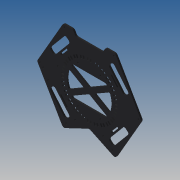
# Autodesk Inventor part: Bottom Plate
Saved by Autodesk Inventor 2017 (Build 210142000, 142)
## iProperties
Created: 2016-10-01
Part Number: Bottom Plate
Material: PVC, Unplasticized
Document SubType Name: Modeling
Designer: James Yelland
Density: 1.29 g/cm^3
Appearance: Smooth - White
Mass: 43.6601 g
Surface Area: 401.333 cm^2
Volume: 33.8451 cm^3
Author: James Yelland
Autodesk Inventor part; units mm, degrees
ref_plane "YZ Plane" through (0, 0, 0) normal (1, 0, 0) x (0, 1, 0)
ref_plane "XZ Plane" through (0, 0, 0) normal (0, 1, 0) x (-1, 0, 0)
ref_plane "XY Plane" through (0, 0, 0) normal (0, 0, 1) x (1, 0, 0)
sketch "Sketch1" plane through (0, 0, 0) normal (0, 1, 0) x (-1, 0, 0)
  line L0 (103.5566, -2.5) -> (54.7862, -86.9325)
  line L1 (-54.8095, -86.9325) -> (-103.5566, -2.5)
  line L2 (-103.5566, 2.5) -> (-53.9434, 88.4327)
  line L3 (53.9434, 88.4327) -> (103.5566, 2.5)
  line L4 (2.1497, -66.9563) -> (48.3064, -88.9468)
  line L5 (-2.1497, -66.9563) -> (-48.3297, -88.9468)
  arc A0 (48.3064, -88.9468) -> (54.7862, -86.9325) centre (50.456, -84.4325) ccw
  arc A1 (2.1497, -66.9563) -> (-2.1497, -66.9563) centre (0, -71.4706) ccw
  arc A2 (-54.8095, -86.9325) -> (-48.3297, -88.9468) centre (-50.4794, -84.4325) ccw
  arc A3 (-103.5566, 2.5) -> (-103.5566, -2.5) centre (-99.2265, 0) ccw
  arc A4 (-49.6132, 90.9327) -> (-53.9434, 88.4327) centre (-49.6132, 85.9327) ccw
  arc A5 (53.9434, 88.4327) -> (49.6132, 90.9327) centre (49.6132, 85.9327) ccw
  arc A6 (103.5566, -2.5) -> (103.5566, 2.5) centre (99.2265, 0) ccw
  circle A7 centre (49.6132, 85.9327) radius 1.6
  circle A8 centre (-49.6132, 85.9327) radius 1.6
  circle A9 centre (-99.2265, 0) radius 1.6
  circle A10 centre (99.2265, 0) radius 1.6
  line L6 (1.5, -53.75) -> (1.5, -56.75)
  line L7 (1.5, -56.75) -> (4.5, -56.75)
  line L8 (4.5, -56.75) -> (4.5, -50.75)
  line L9 (4.5, -50.75) -> (1.5, -50.75)
  line L10 (1.5, -50.75) -> (1.5, -53.75)
  line L11 (-1.5, -53.75) -> (-1.5, -56.75)
  line L12 (-1.5, -56.75) -> (-4.5, -56.75)
  line L13 (-1.5, -53.75) -> (-1.5, -53.75)
  line L14 (-1.5, -53.75) -> (-1.5, -50.75)
  line L15 (-1.5, -50.75) -> (-4.5, -50.75)
  line L16 (-4.5, -56.75) -> (-4.5, -50.75)
  line L17 (15.3604, -51.5303) -> (16.1369, -54.4281)
  line L18 (16.1369, -54.4281) -> (19.0346, -53.6516)
  line L19 (19.0346, -53.6516) -> (17.4817, -47.856)
  line L20 (17.4817, -47.856) -> (14.584, -48.6325)
  line L21 (14.584, -48.6325) -> (15.3604, -51.5303)
  line L22 (12.4626, -52.3067) -> (13.2391, -55.2045)
  line L23 (13.2391, -55.2045) -> (10.3413, -55.981)
  line L24 (12.4626, -52.3067) -> (11.6862, -49.409)
  line L25 (11.6862, -49.409) -> (8.7884, -50.1854)
  line L26 (10.3413, -55.981) -> (8.7884, -50.1854)
  line L27 (28.174, -45.7989) -> (29.674, -48.3969)
  line L28 (29.674, -48.3969) -> (32.2721, -46.8969)
  line L29 (32.2721, -46.8969) -> (29.2721, -41.7008)
  line L30 (29.2721, -41.7008) -> (26.674, -43.2008)
  line L31 (26.674, -43.2008) -> (28.174, -45.7989)
  line L32 (25.576, -47.2989) -> (27.076, -49.8969)
  line L33 (27.076, -49.8969) -> (24.4779, -51.3969)
  line L34 (25.576, -47.2989) -> (24.076, -44.7008)
  line L35 (24.076, -44.7008) -> (21.4779, -46.2008)
  line L36 (24.4779, -51.3969) -> (21.4779, -46.2008)
  line L37 (39.0676, -36.9463) -> (41.189, -39.0676)
  line L38 (41.189, -39.0676) -> (43.3103, -36.9463)
  line L39 (43.3103, -36.9463) -> (39.0676, -32.7037)
  line L40 (39.0676, -32.7037) -> (36.9463, -34.825)
  line L41 (36.9463, -34.825) -> (39.0676, -36.9463)
  line L42 (36.9463, -39.0676) -> (39.0676, -41.189)
  line L43 (39.0676, -41.189) -> (36.9463, -43.3103)
  line L44 (36.9463, -39.0676) -> (34.825, -36.9463)
  line L45 (34.825, -36.9463) -> (32.7037, -39.0676)
  line L46 (36.9463, -43.3103) -> (32.7037, -39.0676)
  line L47 (47.2989, -25.576) -> (49.8969, -27.076)
  line L48 (49.8969, -27.076) -> (51.3969, -24.4779)
  line L49 (51.3969, -24.4779) -> (46.2008, -21.4779)
  line L50 (46.2008, -21.4779) -> (44.7008, -24.076)
  line L51 (44.7008, -24.076) -> (47.2989, -25.576)
  line L52 (45.7989, -28.174) -> (48.3969, -29.674)
  line L53 (48.3969, -29.674) -> (46.8969, -32.2721)
  line L54 (45.7989, -28.174) -> (43.2008, -26.674)
  line L55 (43.2008, -26.674) -> (41.7008, -29.2721)
  line L56 (46.8969, -32.2721) -> (41.7008, -29.2721)
  line L57 (52.3067, -12.4626) -> (55.2045, -13.2391)
  line L58 (55.2045, -13.2391) -> (55.981, -10.3413)
  line L59 (55.981, -10.3413) -> (50.1854, -8.7884)
  line L60 (50.1854, -8.7884) -> (49.409, -11.6862)
  line L61 (49.409, -11.6862) -> (52.3067, -12.4626)
  line L62 (51.5303, -15.3604) -> (54.4281, -16.1369)
  line L63 (54.4281, -16.1369) -> (53.6516, -19.0346)
  line L64 (51.5303, -15.3604) -> (48.6325, -14.584)
  line L65 (48.6325, -14.584) -> (47.856, -17.4817)
  line L66 (53.6516, -19.0346) -> (47.856, -17.4817)
  line L67 (53.75, 1.5) -> (56.75, 1.5)
  line L68 (56.75, 1.5) -> (56.75, 4.5)
  line L69 (56.75, 4.5) -> (50.75, 4.5)
  line L70 (50.75, 4.5) -> (50.75, 1.5)
  line L71 (50.75, 1.5) -> (53.75, 1.5)
  line L72 (53.75, -1.5) -> (56.75, -1.5)
  line L73 (56.75, -1.5) -> (56.75, -4.5)
  line L74 (53.75, -1.5) -> (50.75, -1.5)
  line L75 (50.75, -1.5) -> (50.75, -4.5)
  line L76 (56.75, -4.5) -> (50.75, -4.5)
  line L77 (51.5303, 15.3604) -> (54.4281, 16.1369)
  line L78 (54.4281, 16.1369) -> (53.6516, 19.0346)
  line L79 (53.6516, 19.0346) -> (47.856, 17.4817)
  line L80 (47.856, 17.4817) -> (48.6325, 14.584)
  line L81 (48.6325, 14.584) -> (51.5303, 15.3604)
  line L82 (52.3067, 12.4626) -> (55.2045, 13.2391)
  line L83 (55.2045, 13.2391) -> (55.981, 10.3413)
  line L84 (52.3067, 12.4626) -> (49.409, 11.6862)
  line L85 (49.409, 11.6862) -> (50.1854, 8.7884)
  line L86 (55.981, 10.3413) -> (50.1854, 8.7884)
  line L87 (45.7989, 28.174) -> (48.3969, 29.674)
  line L88 (48.3969, 29.674) -> (46.8969, 32.2721)
  line L89 (46.8969, 32.2721) -> (41.7008, 29.2721)
  line L90 (41.7008, 29.2721) -> (43.2008, 26.674)
  line L91 (43.2008, 26.674) -> (45.7989, 28.174)
  line L92 (47.2989, 25.576) -> (49.8969, 27.076)
  line L93 (49.8969, 27.076) -> (51.3969, 24.4779)
  line L94 (47.2989, 25.576) -> (44.7008, 24.076)
  line L95 (44.7008, 24.076) -> (46.2008, 21.4779)
  line L96 (51.3969, 24.4779) -> (46.2008, 21.4779)
  line L97 (36.9463, 39.0676) -> (39.0676, 41.189)
  line L98 (39.0676, 41.189) -> (36.9463, 43.3103)
  line L99 (36.9463, 43.3103) -> (32.7037, 39.0676)
  line L100 (32.7037, 39.0676) -> (34.825, 36.9463)
  line L101 (34.825, 36.9463) -> (36.9463, 39.0676)
  line L102 (39.0676, 36.9463) -> (41.189, 39.0676)
  line L103 (41.189, 39.0676) -> (43.3103, 36.9463)
  line L104 (39.0676, 36.9463) -> (36.9463, 34.825)
  line L105 (36.9463, 34.825) -> (39.0676, 32.7037)
  line L106 (43.3103, 36.9463) -> (39.0676, 32.7037)
  line L107 (25.576, 47.2989) -> (27.076, 49.8969)
  line L108 (27.076, 49.8969) -> (24.4779, 51.3969)
  line L109 (24.4779, 51.3969) -> (21.4779, 46.2008)
  line L110 (21.4779, 46.2008) -> (24.076, 44.7008)
  line L111 (24.076, 44.7008) -> (25.576, 47.2989)
  line L112 (28.174, 45.7989) -> (29.674, 48.3969)
  line L113 (29.674, 48.3969) -> (32.2721, 46.8969)
  line L114 (28.174, 45.7989) -> (26.674, 43.2008)
  line L115 (26.674, 43.2008) -> (29.2721, 41.7008)
  line L116 (32.2721, 46.8969) -> (29.2721, 41.7008)
  line L117 (12.4626, 52.3067) -> (13.2391, 55.2045)
  line L118 (13.2391, 55.2045) -> (10.3413, 55.981)
  line L119 (10.3413, 55.981) -> (8.7884, 50.1854)
  line L120 (8.7884, 50.1854) -> (11.6862, 49.409)
  line L121 (11.6862, 49.409) -> (12.4626, 52.3067)
  line L122 (15.3604, 51.5303) -> (16.1369, 54.4281)
  line L123 (16.1369, 54.4281) -> (19.0346, 53.6516)
  line L124 (15.3604, 51.5303) -> (14.584, 48.6325)
  line L125 (14.584, 48.6325) -> (17.4817, 47.856)
  line L126 (19.0346, 53.6516) -> (17.4817, 47.856)
  line L127 (-1.5, 53.75) -> (-1.5, 56.75)
  line L128 (-1.5, 56.75) -> (-4.5, 56.75)
  line L129 (-4.5, 56.75) -> (-4.5, 50.75)
  line L130 (-4.5, 50.75) -> (-1.5, 50.75)
  line L131 (-1.5, 50.75) -> (-1.5, 53.75)
  line L132 (1.5, 53.75) -> (1.5, 56.75)
  line L133 (1.5, 56.75) -> (4.5, 56.75)
  line L134 (1.5, 53.75) -> (1.5, 50.75)
  line L135 (1.5, 50.75) -> (4.5, 50.75)
  line L136 (4.5, 56.75) -> (4.5, 50.75)
  line L137 (-15.3604, 51.5303) -> (-16.1369, 54.4281)
  line L138 (-16.1369, 54.4281) -> (-19.0346, 53.6516)
  line L139 (-19.0346, 53.6516) -> (-17.4817, 47.856)
  line L140 (-17.4817, 47.856) -> (-14.584, 48.6325)
  line L141 (-14.584, 48.6325) -> (-15.3604, 51.5303)
  line L142 (-12.4626, 52.3067) -> (-13.2391, 55.2045)
  line L143 (-13.2391, 55.2045) -> (-10.3413, 55.981)
  line L144 (-12.4626, 52.3067) -> (-11.6862, 49.409)
  line L145 (-11.6862, 49.409) -> (-8.7884, 50.1854)
  line L146 (-10.3413, 55.981) -> (-8.7884, 50.1854)
  line L147 (-28.174, 45.7989) -> (-29.674, 48.3969)
  line L148 (-29.674, 48.3969) -> (-32.2721, 46.8969)
  line L149 (-32.2721, 46.8969) -> (-29.2721, 41.7008)
  line L150 (-29.2721, 41.7008) -> (-26.674, 43.2008)
  line L151 (-26.674, 43.2008) -> (-28.174, 45.7989)
  line L152 (-25.576, 47.2989) -> (-27.076, 49.8969)
  line L153 (-27.076, 49.8969) -> (-24.4779, 51.3969)
  line L154 (-25.576, 47.2989) -> (-24.076, 44.7008)
  line L155 (-24.076, 44.7008) -> (-21.4779, 46.2008)
  line L156 (-24.4779, 51.3969) -> (-21.4779, 46.2008)
  line L157 (-39.0676, 36.9463) -> (-41.189, 39.0676)
  line L158 (-41.189, 39.0676) -> (-43.3103, 36.9463)
  line L159 (-43.3103, 36.9463) -> (-39.0676, 32.7037)
  line L160 (-39.0676, 32.7037) -> (-36.9463, 34.825)
  line L161 (-36.9463, 34.825) -> (-39.0676, 36.9463)
  line L162 (-36.9463, 39.0676) -> (-39.0676, 41.189)
  line L163 (-39.0676, 41.189) -> (-36.9463, 43.3103)
  line L164 (-36.9463, 39.0676) -> (-34.825, 36.9463)
  line L165 (-34.825, 36.9463) -> (-32.7037, 39.0676)
  line L166 (-36.9463, 43.3103) -> (-32.7037, 39.0676)
  line L167 (-47.2989, 25.576) -> (-49.8969, 27.076)
  line L168 (-49.8969, 27.076) -> (-51.3969, 24.4779)
  line L169 (-51.3969, 24.4779) -> (-46.2008, 21.4779)
  line L170 (-46.2008, 21.4779) -> (-44.7008, 24.076)
  line L171 (-44.7008, 24.076) -> (-47.2989, 25.576)
  line L172 (-45.7989, 28.174) -> (-48.3969, 29.674)
  line L173 (-48.3969, 29.674) -> (-46.8969, 32.2721)
  line L174 (-45.7989, 28.174) -> (-43.2008, 26.674)
  line L175 (-43.2008, 26.674) -> (-41.7008, 29.2721)
  line L176 (-46.8969, 32.2721) -> (-41.7008, 29.2721)
  line L177 (-52.3067, 12.4626) -> (-55.2045, 13.2391)
  line L178 (-55.2045, 13.2391) -> (-55.981, 10.3413)
  line L179 (-55.981, 10.3413) -> (-50.1854, 8.7884)
  line L180 (-50.1854, 8.7884) -> (-49.409, 11.6862)
  line L181 (-49.409, 11.6862) -> (-52.3067, 12.4626)
  line L182 (-51.5303, 15.3604) -> (-54.4281, 16.1369)
  line L183 (-54.4281, 16.1369) -> (-53.6516, 19.0346)
  line L184 (-51.5303, 15.3604) -> (-48.6325, 14.584)
  line L185 (-48.6325, 14.584) -> (-47.856, 17.4817)
  line L186 (-53.6516, 19.0346) -> (-47.856, 17.4817)
  line L187 (-53.75, -1.5) -> (-56.75, -1.5)
  line L188 (-56.75, -1.5) -> (-56.75, -4.5)
  line L189 (-56.75, -4.5) -> (-50.75, -4.5)
  line L190 (-50.75, -4.5) -> (-50.75, -1.5)
  line L191 (-50.75, -1.5) -> (-53.75, -1.5)
  line L192 (-53.75, 1.5) -> (-56.75, 1.5)
  line L193 (-56.75, 1.5) -> (-56.75, 4.5)
  line L194 (-53.75, 1.5) -> (-50.75, 1.5)
  line L195 (-50.75, 1.5) -> (-50.75, 4.5)
  line L196 (-56.75, 4.5) -> (-50.75, 4.5)
  line L197 (-51.5303, -15.3604) -> (-54.4281, -16.1369)
  line L198 (-54.4281, -16.1369) -> (-53.6516, -19.0346)
  line L199 (-53.6516, -19.0346) -> (-47.856, -17.4817)
  line L200 (-47.856, -17.4817) -> (-48.6325, -14.584)
  line L201 (-48.6325, -14.584) -> (-51.5303, -15.3604)
  line L202 (-52.3067, -12.4626) -> (-55.2045, -13.2391)
  line L203 (-55.2045, -13.2391) -> (-55.981, -10.3413)
  line L204 (-52.3067, -12.4626) -> (-49.409, -11.6862)
  line L205 (-49.409, -11.6862) -> (-50.1854, -8.7884)
  line L206 (-55.981, -10.3413) -> (-50.1854, -8.7884)
  line L207 (-45.7989, -28.174) -> (-48.3969, -29.674)
  line L208 (-48.3969, -29.674) -> (-46.8969, -32.2721)
  line L209 (-46.8969, -32.2721) -> (-41.7008, -29.2721)
  line L210 (-41.7008, -29.2721) -> (-43.2008, -26.674)
  line L211 (-43.2008, -26.674) -> (-45.7989, -28.174)
  line L212 (-47.2989, -25.576) -> (-49.8969, -27.076)
  line L213 (-49.8969, -27.076) -> (-51.3969, -24.4779)
  line L214 (-47.2989, -25.576) -> (-44.7008, -24.076)
  line L215 (-44.7008, -24.076) -> (-46.2008, -21.4779)
  line L216 (-51.3969, -24.4779) -> (-46.2008, -21.4779)
  line L217 (-36.9463, -39.0676) -> (-39.0676, -41.189)
  line L218 (-39.0676, -41.189) -> (-36.9463, -43.3103)
  line L219 (-36.9463, -43.3103) -> (-32.7037, -39.0676)
  line L220 (-32.7037, -39.0676) -> (-34.825, -36.9463)
  line L221 (-34.825, -36.9463) -> (-36.9463, -39.0676)
  line L222 (-39.0676, -36.9463) -> (-41.189, -39.0676)
  line L223 (-41.189, -39.0676) -> (-43.3103, -36.9463)
  line L224 (-39.0676, -36.9463) -> (-36.9463, -34.825)
  line L225 (-36.9463, -34.825) -> (-39.0676, -32.7037)
  line L226 (-43.3103, -36.9463) -> (-39.0676, -32.7037)
  line L227 (-25.576, -47.2989) -> (-27.076, -49.8969)
  line L228 (-27.076, -49.8969) -> (-24.4779, -51.3969)
  line L229 (-24.4779, -51.3969) -> (-21.4779, -46.2008)
  line L230 (-21.4779, -46.2008) -> (-24.076, -44.7008)
  line L231 (-24.076, -44.7008) -> (-25.576, -47.2989)
  line L232 (-28.174, -45.7989) -> (-29.674, -48.3969)
  line L233 (-29.674, -48.3969) -> (-32.2721, -46.8969)
  line L234 (-28.174, -45.7989) -> (-26.674, -43.2008)
  line L235 (-26.674, -43.2008) -> (-29.2721, -41.7008)
  line L236 (-32.2721, -46.8969) -> (-29.2721, -41.7008)
  line L237 (-12.4626, -52.3067) -> (-13.2391, -55.2045)
  line L238 (-13.2391, -55.2045) -> (-10.3413, -55.981)
  line L239 (-10.3413, -55.981) -> (-8.7884, -50.1854)
  line L240 (-8.7884, -50.1854) -> (-11.6862, -49.409)
  line L241 (-11.6862, -49.409) -> (-12.4626, -52.3067)
  line L242 (-15.3604, -51.5303) -> (-16.1369, -54.4281)
  line L243 (-16.1369, -54.4281) -> (-19.0346, -53.6516)
  line L244 (-15.3604, -51.5303) -> (-14.584, -48.6325)
  line L245 (-14.584, -48.6325) -> (-17.4817, -47.856)
  line L246 (-19.0346, -53.6516) -> (-17.4817, -47.856)
  arc A11 (50.7976, 70.0378) -> (45.1623, 70.5308) centre (47.7335, 67.4666) ccw
  line L247 (45.1623, 70.5308) -> (41.3321, 67.3169)
  arc A12 (41.3321, 67.3169) -> (40.8391, 61.6815) centre (43.9032, 64.2527) ccw
  line L248 (64.2962, 53.9509) -> (50.7976, 70.0378)
  line L249 (40.8391, 61.6815) -> (67.8361, 29.5077)
  line L250 (64.2962, 53.9509) -> (77.7947, 37.8639)
  arc A13 (77.3017, 32.2286) -> (77.7947, 37.8639) centre (74.7305, 35.2928) ccw
  line L251 (73.4714, 29.0147) -> (77.3017, 32.2286)
  arc A14 (67.8361, 29.5077) -> (73.4714, 29.0147) centre (70.9003, 32.0789) ccw
  line L252 (0, 30) -> (-31.225, 30)
  line L253 (0, 30) -> (31.225, 30)
  line L254 (0, -30) -> (-31.225, -30)
  line L255 (0, -30) -> (31.225, -30)
  arc A15 (42.1141, -15.8557) -> (42.1141, 15.8557) centre (0, 0) ccw
  arc A16 (-42.1141, 15.8558) -> (-42.1141, -15.8558) centre (0, 0) ccw
  arc A17 (34.525, 28.7563) -> (31.225, 30) centre (31.225, 25) ccw
  arc A18 (-31.225, 30) -> (-34.525, 28.7563) centre (-31.225, 25) ccw
  arc A19 (-34.525, -28.7563) -> (-31.225, -30) centre (-31.225, -25) ccw
  arc A20 (31.225, -30) -> (34.525, -28.7563) centre (31.225, -25) ccw
  circle A21 centre (22.6343, 38) radius 1.6
  circle A22 centre (-22.6343, 38) radius 1.6
  circle A23 centre (-22.6343, -38) radius 1.6
  circle A24 centre (22.6343, -38) radius 1.6
  line L256 (54.3376, 45.5946) -> (57.5515, 41.7644)
  line L257 (39.2424, -16.8831) -> (13, -1.7321)
  line L258 (39.2424, 16.8831) -> (13, 1.7321)
  line L259 (34.205, 25.5218) -> (1, 6.3509)
  line L260 (-1, 6.3509) -> (-34.205, 25.5218)
  line L261 (-39.2423, 16.8832) -> (-12.9998, 1.7321)
  line L262 (-12.9998, -1.7321) -> (-39.2423, -16.8832)
  line L263 (-34.205, -25.5218) -> (-1, -6.3509)
  line L264 (1, -6.3509) -> (34.205, -25.5218)
  arc A25 (-1, 6.3509) -> (1, 6.3509) centre (0, 8.0829) ccw
  arc A26 (-12.9998, -1.7321) -> (-12.9998, 1.7321) centre (-13.9998, 0) ccw
  arc A27 (1, -6.3509) -> (-1, -6.3509) centre (0, -8.0829) ccw
  arc A28 (13, 1.7321) -> (13, -1.7321) centre (14, 0) ccw
  arc A29 (39.2424, -16.8831) -> (42.1141, -15.8557) centre (40.2424, -15.151) ccw
  arc A30 (34.525, -28.7563) -> (34.205, -25.5218) centre (33.205, -27.2538) ccw
  arc A31 (-42.1141, -15.8558) -> (-39.2423, -16.8832) centre (-40.2423, -15.1511) ccw
  arc A32 (-34.205, -25.5218) -> (-34.525, -28.7563) centre (-33.205, -27.2538) ccw
  arc A33 (-39.2423, 16.8832) -> (-42.1141, 15.8558) centre (-40.2423, 15.1511) ccw
  arc A34 (-34.525, 28.7563) -> (-34.205, 25.5218) centre (-33.205, 27.2538) ccw
  arc A35 (42.1141, 15.8557) -> (39.2424, 16.8831) centre (40.2424, 15.151) ccw
  arc A36 (34.205, 25.5218) -> (34.525, 28.7563) centre (33.205, 27.2538) ccw
  line L265 (49.7796, 41.77) -> (43.3517, 49.4305)
  line L266 (43.3517, 49.4305) -> (45.6499, 51.3589)
  line L267 (45.6499, 51.3589) -> (58.5056, 36.038)
  line L268 (58.5056, 36.038) -> (56.2075, 34.1096)
  line L269 (56.2075, 34.1096) -> (49.7796, 41.77)
  arc A37 (73.4714, -29.0147) -> (67.8361, -29.5077) centre (70.9003, -32.0789) ccw
  arc A38 (77.7947, -37.8639) -> (77.3017, -32.2286) centre (74.7305, -35.2928) ccw
  line L270 (73.4714, -29.0147) -> (77.3017, -32.2286)
  arc A39 (45.1623, -70.5308) -> (50.7976, -70.0378) centre (47.7335, -67.4666) ccw
  line L271 (45.1623, -70.5308) -> (41.3321, -67.3169)
  arc A40 (40.8391, -61.6815) -> (41.3321, -67.3169) centre (43.9032, -64.2527) ccw
  line L272 (64.2962, -53.9509) -> (50.7976, -70.0378)
  line L273 (64.2962, -53.9509) -> (77.7947, -37.8639)
  line L274 (40.8391, -61.6815) -> (67.8361, -29.5077)
  line L275 (49.7796, -41.77) -> (43.3517, -49.4305)
  line L276 (43.3517, -49.4305) -> (45.6499, -51.3589)
  line L277 (45.6499, -51.3589) -> (58.5056, -36.038)
  line L278 (58.5056, -36.038) -> (56.2075, -34.1096)
  line L279 (56.2075, -34.1096) -> (49.7796, -41.77)
  arc A41 (-73.4714, 29.0147) -> (-67.8361, 29.5077) centre (-70.9003, 32.0789) ccw
  arc A42 (-77.7947, 37.8639) -> (-77.3017, 32.2286) centre (-74.7305, 35.2928) ccw
  line L280 (-73.4714, 29.0147) -> (-77.3017, 32.2286)
  arc A43 (-45.1623, 70.5308) -> (-50.7976, 70.0378) centre (-47.7335, 67.4666) ccw
  line L281 (-45.1623, 70.5308) -> (-41.3321, 67.3169)
  arc A44 (-40.8391, 61.6815) -> (-41.3321, 67.3169) centre (-43.9032, 64.2527) ccw
  line L282 (-64.2962, 53.9509) -> (-50.7976, 70.0378)
  line L283 (-64.2962, 53.9509) -> (-77.7947, 37.8639)
  line L284 (-40.8391, 61.6815) -> (-67.8361, 29.5077)
  line L285 (-49.7796, 41.77) -> (-43.3517, 49.4305)
  line L286 (-43.3517, 49.4305) -> (-45.6499, 51.3589)
  line L287 (-45.6499, 51.3589) -> (-58.5056, 36.038)
  line L288 (-58.5056, 36.038) -> (-56.2075, 34.1096)
  line L289 (-56.2075, 34.1096) -> (-49.7796, 41.77)
  arc A45 (-67.8361, -29.5077) -> (-73.4714, -29.0147) centre (-70.9003, -32.0789) ccw
  line L290 (-45.6499, -51.3589) -> (-58.5056, -36.038)
  line L291 (-58.5056, -36.038) -> (-56.2075, -34.1096)
  line L292 (-40.8391, -61.6815) -> (-67.8361, -29.5077)
  line L293 (-64.2962, -53.9509) -> (-77.7947, -37.8639)
  line L294 (-73.4714, -29.0147) -> (-77.3017, -32.2286)
  arc A46 (-77.3017, -32.2286) -> (-77.7947, -37.8639) centre (-74.7305, -35.2928) ccw
  line L295 (-43.3517, -49.4305) -> (-45.6499, -51.3589)
  line L296 (-49.7796, -41.77) -> (-43.3517, -49.4305)
  arc A47 (-50.7976, -70.0378) -> (-45.1623, -70.5308) centre (-47.7335, -67.4666) ccw
  line L297 (-64.2962, -53.9509) -> (-50.7976, -70.0378)
  line L298 (-45.1623, -70.5308) -> (-41.3321, -67.3169)
  arc A48 (-41.3321, -67.3169) -> (-40.8391, -61.6815) centre (-43.9032, -64.2527) ccw
  line L299 (-56.2075, -34.1096) -> (-49.7796, -41.77)
  circle A49 centre (28.2679, -64.7457) radius 1.6
  circle A50 centre (-28.2679, -64.7457) radius 1.6
  circle A51 centre (63.1808, 11.5746) radius 1.6
  circle A52 centre (92.6257, -5.4254) radius 1.6
  circle A53 centre (82.6257, -22.7459) radius 1.6
  line L300 (103.5566, -2.5) -> (94.5534, -18.0866)
  line L301 (48.2264, -83.602) -> (48.2264, -77.602)
  line L302 (48.2264, -77.602) -> (45.2264, -77.602)
  line L303 (45.2264, -77.602) -> (45.2264, -83.602)
  line L304 (45.2264, -83.602) -> (48.2264, -83.602)
  line L305 (-48.2265, -83.602) -> (-45.2265, -83.602)
  line L306 (-45.2265, -83.602) -> (-45.2265, -77.602)
  line L307 (-45.2265, -77.602) -> (-48.2265, -77.602)
  line L308 (-48.2265, -77.602) -> (-48.2265, -83.602)
  line L309 (0, 80.9327) -> (24.1132, 80.9327)
  line L310 (28.4434, 83.4327) -> (31.3301, 88.4327)
  line L311 (0, 80.9327) -> (-24.1132, 80.9327)
  line L312 (-28.4434, 83.4327) -> (-31.3301, 88.4327)
  arc A54 (35.6603, 90.9327) -> (31.3301, 88.4327) centre (35.6603, 85.9327) ccw
  arc A55 (-31.3301, 88.4327) -> (-35.6603, 90.9327) centre (-35.6603, 85.9327) ccw
  arc A56 (24.1132, 80.9327) -> (28.4434, 83.4327) centre (24.1132, 85.9327) ccw
  arc A57 (-28.4434, 83.4327) -> (-24.1132, 80.9327) centre (-24.1132, 85.9327) ccw
  line L313 (49.6132, 90.9327) -> (35.6603, 90.9327)
  line L314 (-35.6603, 90.9327) -> (-49.6132, 90.9327)
  point P0 (52.4787, -90.9271)
  point P1 (-52.5, 90.9327)
  point P2 (52.5, 90.9327)
  point P3 (60, 0)
  point P4 (-60, 0)
  point P5 (-60, 0)
  point P6 (38.2679, 64.7457)
  point P7 (48.2265, 73.102)
  point P8 (70.4073, 26.4435)
  point P9 (80.3658, 34.7998)
  point P10 (60, 0)
  point P11 (-33.541, 30)
  point P12 (33.541, 30)
  point P13 (-33.541, -30)
  point P14 (33.541, -30)
  point P15 (41.2298, -18.0305)
  point P16 (41.2298, 18.0305)
  point P17 (-41.2298, 18.0306)
  point P18 (-41.2298, -18.0306)
  point P19 (70.4073, -26.4435)
  point P20 (38.2679, -64.7457)
  point P21 (-70.4073, 26.4435)
  point P22 (-80.3658, 34.7998)
  point P23 (-38.2679, 64.7457)
  point P24 (-48.2265, 73.102)
  point P25 (-70.4073, -26.4435)
  point P26 (-83.093, -27.663)
  point P27 (27, 80.9327)
  point P28 (-27, 80.9327)
  dimension "d11" = 360
  dimension "d30" = 360
  dimension "d114" = 360
  dimension "d174" = 3.2
  dimension "d175" = 3.2
  dimension "d177" = 3.2
  dimension "d178" = 3.2
  dimension "d185" = 6
  dimension "d186" = 27
  dimension "d187" = 120
  dimension "d188" = 27
  dimension "d189" = 120
  dimension "d190" = 5
  dimension "d191" = 5
  constraints: 630 end point, 98 point on circle, 65 point on line, 58 centre point, 6 tangent, 5 equal length, 4 coincident, 2 equal radius, 2 horizontal, 2 perpendicular, 1 midpoint, 1 vertical, 1 other
  measures "d174" diameter of A50
  measures "d175" diameter of A51
  measures "d177" diameter of A52
  measures "d178" diameter of A53
  measures "d185" distance of L306.end L305.end
  measures "d186" distance of L311.start point (27, 80.933)
  measures "d187" angle of L310 L309
  measures "d188" distance of L311.start point (-27, 80.933)
  measures "d189" angle of L311 L312
  measures "d190" radius of A54
  measures "d191" radius of A56
extrude "Extrusion1" add sketch "Sketch1" along normal blind 3.2
body "Solid1"
